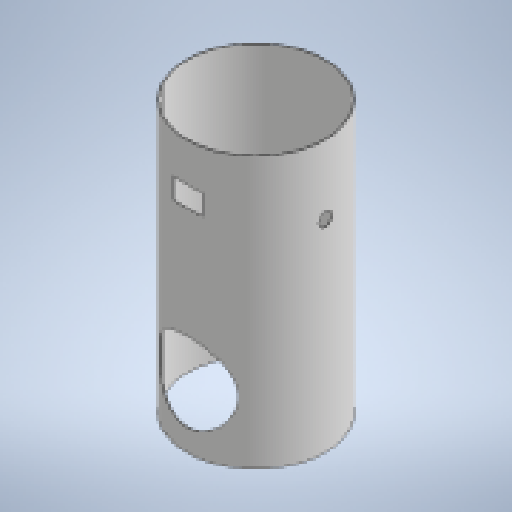
# Autodesk Inventor part: PRS 0101 main shell D1200 940
Saved by Autodesk Inventor 2026.2 (Build 302298000, 298)
## iProperties
Created: 2025-02-11
Part Number: PRS 0101 main shell D1200 940
Material: Steel
Document SubType Name: Sheet Metal
Designer: pokla
Mass: 240408 g
Surface Area: 102828 cm^2
Volume: 30625.3 cm^3
Density: 7.85 g/cm^3
Flat Pattern Width: 183.2 cm
Flat Pattern Length: 293.117 cm
Flat Pattern Area: 53699.1 cm^2
Sheet Metal Rule: Default_mm
Sheet Metal Width: 1832,000 mm
Sheet Metal Length: 2931,171 mm
Sheet Metal Area: 5369905,549 mm^2
Appearance: Default
AA_MAIN_filter_diam: 940,000 mm
Legs_Tube_lenght: 386,705 mm
Legs_Tube_cut_angle: 24,29 grad
Legs_Tube_dim: 80,000 mm
Legs_Upper_plate_lenght: 121,198 mm
Legs_Inner_diam: 676,798 mm
AA_MAIN_Filter_Clearance: 300,000 mm
ChargingHatch_width: 200,000 mm
ChargingHatch_hight: 120,000 mm
AccsessHatch_tube_diameter: 530,000 mm
AA_MAIN_dish_hight: 184,000 mm
Author: pokla
Autodesk Inventor part; units mm, degrees
note: some values were not read from the file. Left out: dimensions or parameters whose unit could not be read.
sketch "Sketch13" plane through (0, 0, 0) normal (0, 0, 1) x (1, 0, 0)
  circle A0 centre (0, 0) radius 470 construction
  line L0 (0, 0) -> (0, -470)
  line L1 (0, 0) -> (-407.0319, -235)
  line L2 (0, 0) -> (470, 0)
  line L3 (0, 0) -> (0, -470)
  line L4 (0, 0) -> (0, -470)
  line L5 (0, 0) -> (418.7731, 213.3755)
  line L6 (0, 0) -> (0, 470)
  dimension "d53" = 940
  dimension "d55" = 0
  dimension "d98" = 180
  dimension "d99" = 240
  dimension "d100" = 63
  dimension "d101" = 90
  constraints: 14 end point, 1 coincident, 1 point on line, 1 vertical, 9 other
  measures "d55" distance between parallel lines of L0 L4
  measures "d98" angle of L3 L6
  measures "d100" angle of L6 L5
  measures "d101" angle of L2 L6
ref_plane "WeldJoint" through (0, 0, -10) normal (0.5, -0.866, 0) x (0, 0, 1)
ref_plane "Inlet_Clock_Angle_plane" through (0, 0, -10) normal (0, 1, 0) x (0, 0, 1)
ref_plane "Charging" through (0, 0, -10) normal (1, 0, 0) x (0, 0, 1)
ref_plane "Accsess" through (0, 0, -10) normal (1, 0, 0) x (0, 0, 1)
sketch "Sketch14" plane through (0, 0, -10) normal (0.5, -0.866, 0) x (0, 0, 1)
  line L0 (1842, 464) -> (10, 464)
  line L1 (10, 464) -> (10, 470)
  line L2 (10, 470) -> (1842, 470)
  line L3 (1842, 470) -> (1842, 464)
  line L4 (10, 0) -> (1842, 0)
  line L5 (10, 470) -> (-20, 470) construction
  line L6 (10, 464) -> (-20, 464) construction
  arc A0 (-20, 464) -> (-74.1579, 429.8249) centre (-20, 404) ccw construction
  arc A1 (-74.1579, 429.8249) -> (-168, 15) centre (795.7784, 15) ccw construction
  line L7 (-168, 15) -> (-168, 0) construction
  line L8 (10, 0) -> (-168, 0) construction
  arc A2 (-20, 470) -> (-79.5736, 432.4074) centre (-20, 404) ccw construction
  arc A3 (-79.5736, 432.4074) -> (-174, 15) centre (795.7784, 15) ccw construction
  line L9 (-174, 15) -> (-174, 0) construction
  line L10 (-168, 0) -> (-174, 0) construction
  line L11 (1842, 464) -> (1872, 464)
  line L12 (1842, 470) -> (1872, 470)
  line L13 (1842, 0) -> (2020, 0) construction
  line L14 (2026, 0) -> (2026, 15) construction
  arc A4 (2026, 15) -> (1931.5736, 432.4074) centre (1056.2216, 15) ccw construction
  arc A5 (1931.5736, 432.4074) -> (1872, 470) centre (1872, 404) ccw construction
  line L15 (2020, 0) -> (2020, 15) construction
  line L16 (2020, 0) -> (2026, 0) construction
  arc A6 (2020, 15) -> (1926.1579, 429.8249) centre (1056.2216, 15) ccw construction
  arc A7 (1926.1579, 429.8249) -> (1872, 464) centre (1872, 404) ccw construction
  line L17 (-119.3891, 418.399) -> (-474, 418.399)
  line L18 (-474, 418.399) -> (-474, 338.399)
  line L19 (-474, 338.399) -> (-119.3891, 338.399)
  line L20 (-119.3891, 338.399) -> (-119.3891, 418.399)
  line L21 (2026, 15) -> (2056, 15) construction
  line L22 (2056, 15) -> (2056, 0) construction
  line L23 (2056, 0) -> (2026, 0) construction
  line L24 (-474, 498.399) -> (-474, 418.399)
  line L25 (-474, 498.399) -> (-468, 498.399)
  line L26 (-468, 498.399) -> (-468, 418.399)
  line L27 (-81.71, 432.3205) -> (-126.8357, 319.837)
  line L28 (-119.3891, 418.399) -> (-87.295, 418.399)
  line L29 (-74.1579, 429.8249) -> (-79.5736, 432.4074)
  line L30 (-81.71, 432.3205) -> (-81.3377, 433.2486) construction
  line L31 (-81.3377, 433.2486) -> (-79.5736, 432.4074) construction
  line L32 (-474, 498.399) -> (-474, 498.399)
  line L33 (-474, 498.399) -> (-474, 338.399)
  line L34 (-474, 338.399) -> (-474, 338.399)
  line L35 (1421, 470) -> (1331, 470)
  line L36 (1331, 470) -> (1331, 570)
  line L37 (1331, 570) -> (1421, 570)
  line L38 (1421, 570) -> (1421, 470)
  point P0 (10, 467)
  point P1 (-104.2729, 376.0787)
  point P2 (1376, 570)
  dimension "d59" = 1832
  dimension "d60" = 6
  dimension "d61" = 940
  dimension "d82" = 60
  dimension "d83" = 30
  dimension "d86" = 80
  dimension "d87" = 30
  dimension "d91" = 15
  dimension "d92" = 20
  dimension "d93" = 184
  dimension "d94" = 30
  dimension "d103" = 386.705
  dimension "d104" = 21.86
  dimension "d105" = 121.1976
  dimension "d107" = 1
  dimension "d108" = 676.798
  dimension "d109" = 0
  dimension "d110" = 2530
  dimension "d111" = 300
  dimension "d112" = 100
  dimension "d113" = 90
  dimension "d114" = 1850
  dimension "d115" = 1366
  constraints: 78 end point, 18 point on circle, 14 horizontal, 13 tangent, 10 perpendicular, 8 centre point, 7 point on line, 6 equal length, 6 parallel, 4 concentric, 3 midpoint, 2 collinear, 2 equal radius, 2 vertical, 1 vertical alignment
  measures "d59" distance of L1.end L2.end
  measures "d60" distance of L0.end L1.end
  measures "d61" diameter of L2 L4
  measures "d82" radius of A0
  measures "d83" distance of L0.end L6.end
  measures "d86" distance of L17.end L18.end
  measures "d87" distance of L14.end L21.end
  measures "d91" distance of L28.end L27.start
  measures "d92" distance of L19.end L27.end
  measures "d93" distance of L9.end L4.start
  measures "d94" diameter of L9.start L4
  measures "d103" distance from line of L18 L28.end
  measures "d104" angle of L20 L27
  measures "d105" distance of L27.end L27.start
  measures "d107" distance of L27.start L30.end
  measures "d108" diameter of L19 L4
  measures "d109" distance of L24.start L32.end
  measures "d110" distance between parallel lines of L33 L22
  measures "d111" distance between parallel lines of L9 L33
  measures "d112" distance of L37.end L35.start
  measures "d113" distance of L36.end L37.end
  measures "d114" distance from line of L33 point (1376, 570)
  measures "d115" distance from line of L1 point (1376, 570)
revolve "Revolution2" add sketch "Sketch14" angle 359.9 about axis through (0, 0, 0) along (0, 0, 1) contours L0 L1 L2 L3
sketch "Sketch AnglePlane_InletPipe" plane through (0, 0, -10) normal (0, 1, 0) x (0, 0, 1)
  line L0 (10, -470) -> (10, 470) projected
  line L1 (10, 0) -> (1376, 0)
  line L2 (1376, 0) -> (1376, 470)
  line L3 (1376, 470) -> (10, 470)
  line L4 (10, 470) -> (10, 0)
  point P0 (10, -407.0319)
  point P1 (10, -407.4415)
  dimension "d63" = 940
  dimension "d64" = 90
  dimension "frd_hght" = 1366
  constraints: 8 end point, 1 collinear, 1 horizontal, 1 parallel
  measures "d63" diameter of L3 L1
  measures "d64" angle of L2 L3
  measures "frd_hght" distance of L2.end L3.end
ref_plane "InletPipe_AnglePlane" through (0, 0, 1366) normal (1, 0, 0) x (0, 1, 0)
sketch "Sketch16" plane through (0, 0, 1366) normal (1, 0, 0) x (0, 1, 0)
  circle A0 centre (0, 0) radius 45.5
  point P0 (0, -1366)
  point P1 (0, 0)
  point P2 (0, 0)
  point P3 (0, 0)
  dimension "d66" = 91
  constraints: 1 centre point, 1 coincident
  measures "d66" diameter of A0
extrude "Extrusion7" cut sketch "Sketch16" along normal through all
ref_plane "Work Plane16" through (0, 0, 0) normal (0, -1, 0) x (1, 0, 0)
sketch "Sketch17" plane through (0, 0, 0) normal (0, -1, 0) x (1, 0, 0)
  circle A0 centre (0, 417.5) radius 267.5
  line L0 (0, 150) -> (-495.5727, 150)
  point P0 (0, 0)
  dimension "d69" = 535
  dimension "d71" = 150
  constraints: 2 end point, 2 horizontal, 2 vertical alignment, 2 other
  measures "d71" distance from line of point (0, 0) L0
extrude "Extrusion8" cut sketch "Sketch17" along normal through all
sketch "ChargingAngleSketch19" plane through (0, 0, -10) normal (1, 0, 0) x (0, 0, 1)
  line L0 (10, 0) -> (1170.6454, 0)
  line L1 (1170.6454, 0) -> (1442, 470)
  line L2 (1442, 470) -> (10, 470)
  line L3 (10, 470) -> (10, 0)
  dimension "d74" = 1432
  dimension "d76" = 940
  dimension "d77" = 60
  constraints: 8 end point, 1 horizontal, 1 parallel, 1 perpendicular
  measures "d74" distance of L1.end L2.end
  measures "d76" diameter of L2 L0
  measures "d77" angle of L2 L1
ref_plane "Work Plane18" through (0, 0, 1160.6454) normal (0, -0.866, 0.5) x (1, 0, 0)
sketch "Sketch20" plane through (0, 0, 1160.6454) normal (0, -0.866, 0.5) x (1, 0, 0)
  line L0 (-100, 0) -> (100, 0)
  line L1 (100, 0) -> (100, 120)
  line L2 (100, 120) -> (-100, 120)
  line L3 (-100, 120) -> (-100, 0)
  point P0 (0, -1005.1484)
  point P1 (0, 0)
  point P2 (0, 0)
  point P3 (0, 0)
  point P4 (0, 0)
  dimension "d78" = 200
  dimension "d79" = 120
  constraints: 8 end point, 2 parallel, 1 coincident, 1 horizontal, 1 midpoint, 1 perpendicular
  measures "d78" distance of L2.end L1.end
  measures "d79" distance of L1.end L0.end
extrude "Charging hole" cut sketch "Sketch20" along normal through all
equation "\"BendRadius\" = Thickness"
equation "\"BendReliefWidth\" = Thickness"
equation "\"BendReliefDepth\" = 0.5 * Thickness"
equation "\"CornerReliefSize\" = 4 * Thickness"
equation "\"MinimumRemnant\" = 2 * Thickness"
equation "\"TransitionRadius\" = BendRadius"
equation "\"JacobiRadiusSize\" = BendRadius"
equation "\"GapSize\" = Thickness"
equation "\"InletPipe_horisont_angle\" = 0"
equation "\"AccsessHatch_ClockAngle\" = 0"
equation "\"ChargingHatch_ClockAgnle\" = 180deg"
equation "\"InletPipe_Clock_angle\" = 90deg"
equation "\"OutletPipe_ClockAngle\" = 63deg"
equation "\"WeldJoint_ClockAgnle\" = 240deg"
equation "\"AA_MAIN_Shell_hight\" = 1832"
equation "\"Legs_Tube_lenght\" = 386.70499"
equation "\"Legs_Upper_plate_lenght\" = 121.19761"
equation "\"Legs_Inner_diam\" = 676.79799"
equation "\"AA_MAIN_dish_hight\" = 184"
equation "\"Thickness\" = 6"
body "Solid2"
